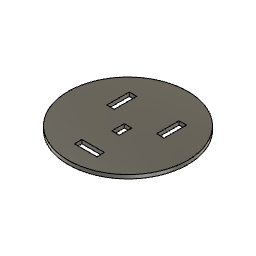
face (Autodesk Fusion 360 design; units mm, degrees)
Autodesk Fusion 360 part; units mm, degrees
sketch "Sketch1" plane through (0, 0, 0) normal (0, 0, 1) x (1, 0, 0)
  circle A0 centre (0, 0) radius 48
  line L0 (9, -34) -> (-9, -34)
  line L1 (-9, -34) -> (-9, -28)
  line L2 (-9, -28) -> (9, -28)
  line L3 (9, -28) -> (9, -34)
  line L4 (9, -34) -> (-9, -28) construction
  line L5 (-9, -34) -> (9, -28) construction
  line L6 (3, -10) -> (-3, -10)
  line L7 (-3, -10) -> (-3, 0)
  line L8 (-3, 0) -> (3, 0)
  line L9 (3, 0) -> (3, -10)
  line L10 (3, -10) -> (-3, 0) construction
  line L11 (-3, -10) -> (3, 0) construction
  line L12 (-17, 6) -> (-23, 6)
  line L13 (-23, 6) -> (-23, 24)
  line L14 (-23, 24) -> (-17, 24)
  line L15 (-17, 24) -> (-17, 6)
  line L16 (-17, 6) -> (-23, 24) construction
  line L17 (-23, 6) -> (-17, 24) construction
  line L18 (23, 6) -> (17, 6)
  line L19 (17, 6) -> (17, 24)
  line L20 (17, 24) -> (23, 24)
  line L21 (23, 24) -> (23, 6)
  line L22 (23, 6) -> (17, 24) construction
  line L23 (17, 6) -> (23, 24) construction
  line L24 (0, -48) -> (0, 48) construction
  line L25 (-20, 15) -> (20, 15) construction
  point P0 (0, -31)
  point P1 (-20, 15)
  point P2 (0, -5)
  point P3 (20, 15)
  point P4 (0, -31)
  point P5 (0, -5)
  point P6 (-20, 15)
  point P7 (20, 15)
  point P8 (0, 15)
  dimension "d1" = 96
  dimension "d2" = 18
  dimension "d3" = 6
  dimension "d4" = 10
  dimension "d5" = 6
  dimension "d6" = 18
  dimension "d7" = 6
  dimension "d8" = 18
  dimension "d9" = 6
  dimension "d12" = 31
  dimension "d13" = 40
  dimension "d14" = 15
  constraint coincident A0.centre origin
  constraint perpendicular L0 L1
  constraint parallel L0 L2
  constraint parallel L1 L3
  constraint horizontal L0
  constraint coincident L4 P4
  constraint coincident L5 P4
  constraint coincident P4 P0
  constraint perpendicular L6 L7
  constraint parallel L6 L8
  constraint parallel L7 L9
  constraint horizontal L6
  constraint coincident L10 P5
  constraint coincident L11 P5
  constraint coincident P5 P2
  constraint perpendicular L12 L13
  constraint parallel L12 L14
  constraint parallel L13 L15
  constraint horizontal L12
  constraint coincident L16 P6
  constraint coincident L17 P6
  constraint coincident P6 P1
  constraint perpendicular L18 L19
  constraint parallel L18 L20
  constraint parallel L19 L21
  constraint horizontal L18
  constraint coincident L22 P7
  constraint coincident L23 P7
  constraint coincident P7 P3
  constraint coincident A0.centre L8
  constraint coincident A0 L24.start
  constraint coincident A0 L24.end
  constraint vertical L24
  constraint coincident A0.centre L24
  constraint coincident P5 L24
  constraint coincident P4 L24
  constraint perpendicular L19 L25
  constraint coincident L25 P8
  constraint coincident L24 P8
  constraint midpoint L25 P8
  measures "d1" diameter of A0
  measures "d2" distance of L1.end L2.end
  measures "d3" distance of L0.end L1.end
  measures "d4" distance of L6.end L7.end
  measures "d5" distance of L7.end L8.end
  measures "d6" distance of L12.end L13.end
  measures "d7" distance of L13.end L14.end
  measures "d8" distance of L18.end L19.end
  measures "d9" distance of L19.end L20.end
  measures "d12" distance of A0.centre P4
  measures "d13" distance of P6 P7
  measures "d14" distance of A0.centre P8
extrude "Extrude3" add sketch "Sketch1" along normal blind 3
